Autodesk Inventor part; units mm, degrees
(part 2 of 2)
sketch "Sketch3" plane through (0, 2, 0) normal (0, 1, 0) x (1, 0, 0)
  arc A0 (-46.6476, -62.1619) -> (-47.7526, -62.2283) centre (-47.0018, -65.4919) ccw
  line L0 (-47.7526, -62.2283) -> (-47.7526, -54.9637)
  arc A1 (-46.6476, -56.7523) -> (-47.7526, -54.9637) centre (-48.6476, -56.7523) ccw
  line L1 (-46.1538, -36) -> (-46.1538, -63.7839)
  line L2 (-57.0002, -27.1688) -> (-56.9998, -63.0741)
  line L3 (-56.9998, -63.0741) -> (-59.9998, -63.0742)
  line L4 (-59.9998, -63.0742) -> (-59.9995, -79.762)
  line L5 (-59.9995, -79.762) -> (-57.0005, -79.762)
  line L6 (-57.0005, -79.762) -> (-57.0005, -94.8331)
  line L7 (-57.0005, -94.8331) -> (-41.6794, -94.8331)
  line L8 (-41.6794, -94.8331) -> (-41.6794, -97.8331)
  line L9 (-41.6794, -97.8331) -> (-24.9903, -97.8331)
  line L10 (-24.9903, -97.8331) -> (-24.9903, -94.8331)
  line L11 (-24.9903, -94.8331) -> (24.9903, -94.8331)
  line L12 (24.9903, -94.8331) -> (24.9903, -97.8331)
  line L13 (24.9903, -97.8331) -> (41.6794, -97.8331)
  line L14 (41.6794, -97.8331) -> (41.6794, -94.8331)
  line L15 (41.6794, -94.8331) -> (57.0005, -94.8331)
  line L16 (57.0005, -94.8331) -> (57.0005, -79.762)
  line L17 (57.0005, -79.762) -> (60.0005, -79.762)
  line L18 (60.0005, -79.762) -> (60.0005, -63.0729)
  line L19 (60.0005, -63.0729) -> (57.0005, -63.0729)
  line L20 (57.0005, -63.0729) -> (57.0002, -27.1688)
  line L21 (57.0002, -27.1688) -> (-57.0002, -27.1688)
  circle A2 centre (-10.4999, -30.1712) radius 1
  circle A3 centre (10.5001, -30.1708) radius 1
  circle A4 centre (23.9057, -30.1706) radius 1
  circle A5 centre (44.9057, -30.1702) radius 1
  circle A6 centre (-23.9063, -30.1714) radius 1
  circle A7 centre (-44.9063, -30.1718) radius 1
  circle A8 centre (-47.0018, -34.2919) radius 1.75
  circle A9 centre (28.1782, -34.2919) radius 1.75
  circle A10 centre (28.1782, -65.4919) radius 1.75
  circle A11 centre (-47.0018, -65.4919) radius 1.75
  circle A12 centre (-35.535, -80.373) radius 1.75
  circle A13 centre (34.465, -80.373) radius 1.75
  circle A14 centre (-6.604, -75.238) radius 3
  circle A15 centre (6.604, -75.238) radius 3
  circle A16 centre (-21.844, -75.746) radius 6.43
  circle A17 centre (21.844, -75.746) radius 6.43
  arc A18 (-46.6476, -56.7523) -> (-47.7526, -54.9637) centre (-48.6476, -56.7523) ccw
  line L22 (-46.6476, -56.7523) -> (-46.6476, -62.1619)
  arc A19 (-46.6476, -62.1619) -> (-47.7526, -62.2283) centre (-47.0018, -65.4919) ccw
  line L23 (-46.6476, -68.822) -> (-46.6476, -85.7402)
  arc A20 (-48.6476, -87.7402) -> (-46.6476, -85.7402) centre (-48.6476, -85.7402) ccw
  line L24 (-48.6476, -87.7402) -> (-50.6476, -87.7402)
  arc A21 (-52.6476, -85.7402) -> (-50.6476, -87.7402) centre (-50.6476, -85.7402) ccw
  arc A22 (50.6476, -87.7402) -> (52.6476, -85.7402) centre (50.6476, -85.7402) ccw
  line L25 (50.6476, -87.7402) -> (48.6476, -87.7402)
  arc A23 (46.6476, -85.7402) -> (48.6476, -87.7402) centre (48.6476, -85.7402) ccw
  line L26 (46.6476, -85.7402) -> (46.6476, -56.7523)
  arc A24 (48.6476, -54.7523) -> (46.6476, -56.7523) centre (48.6476, -56.7523) ccw
  line L27 (48.6476, -54.7523) -> (50.6476, -54.7523)
  arc A25 (52.6476, -56.7523) -> (50.6476, -54.7523) centre (50.6476, -56.7523) ccw
  line L28 (52.6476, -56.7523) -> (52.6476, -85.7402)
  line L29 (27.3301, -36) -> (27.3301, -63.7839)
  line L30 (27.3301, -63.7839) -> (-46.1538, -63.7839)
  line L31 (-46.1538, -63.7839) -> (-46.1538, -36)
  line L32 (-46.1538, -36) -> (27.3301, -36)
  line L33 (38.2149, -69.0614) -> (37.21, -69.0614)
  line L34 (37.21, -69.0614) -> (37.21, -65.8232)
  line L35 (37.21, -65.8232) -> (36.0269, -65.8232)
  line L36 (36.0269, -65.8232) -> (36.0269, -65.0614)
  line L37 (36.0269, -65.0614) -> (39.398, -65.0614)
  line L38 (39.398, -65.0614) -> (39.398, -65.8232)
  line L39 (39.398, -65.8232) -> (38.2149, -65.8232)
  line L40 (38.2149, -65.8232) -> (38.2149, -69.0614)
  spline S0 degree 2 poles (39.3883, -54.4407) (39.3883, -55.1798) (38.5423, -55.9739) (37.7124, -55.9739) knots 0 0 0 1 2 2 2
  spline S1 degree 2 poles (37.7124, -55.9739) (36.9053, -55.9739) (36.0366, -55.196) (36.0366, -54.4439) knots 0 0 0 1 2 2 2
  line L41 (36.0366, -54.4439) -> (36.0366, -51.8896)
  line L42 (36.0366, -51.8896) -> (37.0415, -51.8896)
  line L43 (37.0415, -51.8896) -> (37.0415, -54.3856)
  spline S2 degree 2 poles (37.0415, -54.3856) (37.0415, -54.8037) (37.3559, -55.2122) (37.7124, -55.2122) knots 0 0 0 1 2 2 2
  spline S3 degree 2 poles (37.7124, -55.2122) (38.0593, -55.2122) (38.3834, -54.8199) (38.3834, -54.3856) knots 0 0 0 1 2 2 2
  line L44 (38.3834, -54.3856) -> (38.3834, -51.8896)
  line L45 (38.3834, -51.8896) -> (39.3883, -51.8896)
  line L46 (39.3883, -51.8896) -> (39.3883, -54.4407)
  line L47 (32.7825, -86.0448) -> (32.7825, -86.9605)
  line L48 (32.7825, -86.9605) -> (31.5385, -86.9605)
  line L49 (31.5385, -86.9605) -> (31.5385, -86.0448)
  line L50 (31.5385, -86.0448) -> (32.7825, -86.0448)
  spline S4 degree 2 poles (30.5337, -91.0002) (30.2946, -91.1785) (29.6382, -91.373) (29.1803, -91.373) knots 0 0 0 1 2 2 2
  spline S5 degree 2 poles (29.1803, -91.373) (28.7671, -91.373) (28.0256, -91.1906) (27.7825, -91.0691) knots 0 0 0 1 2 2 2
  line L51 (27.7825, -91.0691) -> (27.7825, -90.0764)
  line L52 (27.7825, -90.0764) -> (27.8797, -90.0764)
  spline S6 degree 2 poles (27.8797, -90.0764) (27.9648, -90.1412) (28.1795, -90.2952) (28.37, -90.3803) knots 0 0 0 1 2 2 2
  spline S7 degree 2 poles (28.37, -90.3803) (28.5361, -90.4573) (28.9453, -90.5667) (29.1885, -90.5667) knots 0 0 0 1 2 2 2
  spline S8 degree 2 poles (29.1885, -90.5667) (29.4356, -90.5667) (29.8165, -90.4127) (29.8165, -90.2466) knots 0 0 0 1 2 2 2
  spline S9 degree 2 poles (29.8165, -90.2466) (29.8165, -90.1169) (29.6423, -89.9791) (29.391, -89.9224) knots 0 0 0 1 2 2 2
  spline S10 degree 2 poles (29.391, -89.9224) (29.2573, -89.8859) (28.8481, -89.809) (28.6901, -89.7603) knots 0 0 0 1 2 2 2
  spline S11 degree 2 poles (28.6901, -89.7603) (28.2444, -89.6226) (27.7987, -89.0837) (27.7987, -88.642) knots 0 0 0 1 2 2 2
  spline S12 degree 2 poles (27.7987, -88.642) (27.7987, -88.3908) (28.0296, -87.9451) (28.2565, -87.7709) knots 0 0 0 1 2 2 2
  spline S13 degree 2 poles (28.2565, -87.7709) (28.4794, -87.6007) (29.1398, -87.3981) (29.5572, -87.3981) knots 0 0 0 1 2 2 2
  spline S14 degree 2 poles (29.5572, -87.3981) (29.9543, -87.3981) (30.6188, -87.5561) (30.8457, -87.6655) knots 0 0 0 1 2 2 2
  line L53 (30.8457, -87.6655) -> (30.8457, -88.6218)
  line L54 (30.8457, -88.6218) -> (30.7525, -88.6218)
  spline S15 degree 2 poles (30.7525, -88.6218) (30.6917, -88.5731) (30.4283, -88.4151) (30.3068, -88.3584) knots 0 0 0 1 2 2 2
  spline S16 degree 2 poles (30.3068, -88.3584) (30.1568, -88.2936) (29.7922, -88.2044) (29.6017, -88.2044) knots 0 0 0 1 2 2 2
  spline S17 degree 2 poles (29.6017, -88.2044) (29.3465, -88.2044) (28.994, -88.3786) (28.994, -88.5205) knots 0 0 0 1 2 2 2
  spline S18 degree 2 poles (28.994, -88.5205) (28.994, -88.6501) (29.1682, -88.796) (29.4599, -88.8689) knots 0 0 0 1 2 2 2
  spline S19 degree 2 poles (29.4599, -88.8689) (29.6098, -88.9054) (30.0029, -88.9743) (30.1852, -89.035) knots 0 0 0 1 2 2 2
  spline S20 degree 2 poles (30.1852, -89.035) (30.5904, -89.1647) (31.0118, -89.6712) (31.0118, -90.0926) knots 0 0 0 1 2 2 2
  spline S21 degree 2 poles (31.0118, -90.0926) (31.0118, -90.356) (30.7646, -90.8381) (30.5337, -91.0002) knots 0 0 0 1 2 2 2
  spline S22 degree 2 poles (26.7695, -91.2636) (26.5791, -91.3162) (26.1739, -91.373) (25.8821, -91.373) knots 0 0 0 1 2 2 2
  spline S23 degree 2 poles (25.8821, -91.373) (24.8124, -91.373) (23.6739, -90.3519) (23.6739, -89.4078) knots 0 0 0 1 2 2 2
  spline S24 degree 2 poles (23.6739, -89.4078) (23.6739, -88.484) (24.7355, -87.3819) (25.6917, -87.3819) knots 0 0 0 1 2 2 2
  spline S25 degree 2 poles (25.6917, -87.3819) (26.5547, -87.3819) (27.4299, -88.3179) (27.4299, -89.185) knots 0 0 0 1 2 2 2
  line L55 (27.4299, -89.185) -> (27.4299, -89.6104)
  line L56 (27.4299, -89.6104) -> (24.8489, -89.6104)
  spline S26 degree 2 poles (24.8489, -89.6104) (24.8651, -89.8738) (25.0555, -90.2222) (25.2095, -90.3276) knots 0 0 0 1 2 2 2
  spline S27 degree 2 poles (25.2095, -90.3276) (25.3594, -90.4329) (25.7646, -90.5221) (26.0037, -90.5221) knots 0 0 0 1 2 2 2
  spline S28 degree 2 poles (26.0037, -90.5221) (26.2063, -90.5221) (26.6034, -90.4329) (26.7695, -90.356) knots 0 0 0 1 2 2 2
  spline S29 degree 2 poles (26.7695, -90.356) (26.9154, -90.2952) (27.1585, -90.1453) (27.2355, -90.0885) knots 0 0 0 1 2 2 2
  line L57 (27.2355, -90.0885) -> (27.3611, -90.0885)
  line L58 (27.3611, -90.0885) -> (27.3611, -91.061)
  spline S30 degree 2 poles (27.3611, -91.061) (27.2152, -91.1177) (26.9802, -91.215) (26.7695, -91.2636) knots 0 0 0 1 2 2 2
  line L59 (10.1082, -88.8162) -> (10.1082, -91.2717)
  line L60 (10.1082, -91.2717) -> (8.9251, -91.2717)
  line L61 (8.9251, -91.2717) -> (8.9251, -89.4038)
  spline S31 degree 2 poles (8.9251, -89.4038) (8.9251, -89.1728) (8.8886, -88.719) (8.84, -88.6137) knots 0 0 0 1 2 2 2
  spline S32 degree 2 poles (8.84, -88.6137) (8.7792, -88.484) (8.5523, -88.3746) (8.3578, -88.3746) knots 0 0 0 1 2 2 2
  spline S33 degree 2 poles (8.3578, -88.3746) (8.216, -88.3746) (7.9202, -88.484) (7.7541, -88.6015) knots 0 0 0 1 2 2 2
  line L62 (7.7541, -88.6015) -> (7.7541, -91.2717)
  line L63 (7.7541, -91.2717) -> (6.5791, -91.2717)
  line L64 (6.5791, -91.2717) -> (6.5791, -87.4994)
  line L65 (6.5791, -87.4994) -> (7.7541, -87.4994)
  line L66 (7.7541, -87.4994) -> (7.7541, -87.9167)
  spline S34 degree 2 poles (7.7541, -87.9167) (8.0418, -87.6736) (8.5888, -87.3981) (8.921, -87.3981) knots 0 0 0 1 2 2 2
  spline S35 degree 2 poles (8.921, -87.3981) (9.4964, -87.3981) (10.1082, -88.1274) (10.1082, -88.8162) knots 0 0 0 1 2 2 2
  spline S36 degree 2 poles (0.2055, -91.0002) (-0.0336, -91.1785) (-0.69, -91.373) (-1.1479, -91.373) knots 0 0 0 1 2 2 2
  spline S37 degree 2 poles (-1.1479, -91.373) (-1.5611, -91.373) (-2.3026, -91.1906) (-2.5457, -91.0691) knots 0 0 0 1 2 2 2
  line L67 (-2.5457, -91.0691) -> (-2.5457, -90.0764)
  line L68 (-2.5457, -90.0764) -> (-2.4485, -90.0764)
  spline S38 degree 2 poles (-2.4485, -90.0764) (-2.3634, -90.1412) (-2.1487, -90.2952) (-1.9582, -90.3803) knots 0 0 0 1 2 2 2
  spline S39 degree 2 poles (-1.9582, -90.3803) (-1.7921, -90.4573) (-1.3829, -90.5667) (-1.1398, -90.5667) knots 0 0 0 1 2 2 2
  spline S40 degree 2 poles (-1.1398, -90.5667) (-0.8926, -90.5667) (-0.5117, -90.4127) (-0.5117, -90.2466) knots 0 0 0 1 2 2 2
  spline S41 degree 2 poles (-0.5117, -90.2466) (-0.5117, -90.1169) (-0.6859, -89.9791) (-0.9372, -89.9224) knots 0 0 0 1 2 2 2
  spline S42 degree 2 poles (-0.9372, -89.9224) (-1.0709, -89.8859) (-1.4801, -89.809) (-1.6381, -89.7603) knots 0 0 0 1 2 2 2
  spline S43 degree 2 poles (-1.6381, -89.7603) (-2.0838, -89.6226) (-2.5295, -89.0837) (-2.5295, -88.642) knots 0 0 0 1 2 2 2
  spline S44 degree 2 poles (-2.5295, -88.642) (-2.5295, -88.3908) (-2.2986, -87.9451) (-2.0717, -87.7709) knots 0 0 0 1 2 2 2
  spline S45 degree 2 poles (-2.0717, -87.7709) (-1.8488, -87.6007) (-1.1884, -87.3981) (-0.771, -87.3981) knots 0 0 0 1 2 2 2
  spline S46 degree 2 poles (-0.771, -87.3981) (-0.3739, -87.3981) (0.2906, -87.5561) (0.5175, -87.6655) knots 0 0 0 1 2 2 2
  line L69 (0.5175, -87.6655) -> (0.5175, -88.6218)
  line L70 (0.5175, -88.6218) -> (0.4243, -88.6218)
  spline S47 degree 2 poles (0.4243, -88.6218) (0.3635, -88.5731) (0.1001, -88.4151) (-0.0214, -88.3584) knots 0 0 0 1 2 2 2
  spline S48 degree 2 poles (-0.0214, -88.3584) (-0.1714, -88.2936) (-0.536, -88.2044) (-0.7265, -88.2044) knots 0 0 0 1 2 2 2
  spline S49 degree 2 poles (-0.7265, -88.2044) (-0.9817, -88.2044) (-1.3342, -88.3786) (-1.3342, -88.5205) knots 0 0 0 1 2 2 2
  spline S50 degree 2 poles (-1.3342, -88.5205) (-1.3342, -88.6501) (-1.16, -88.796) (-0.8683, -88.8689) knots 0 0 0 1 2 2 2
  spline S51 degree 2 poles (-0.8683, -88.8689) (-0.7184, -88.9054) (-0.3253, -88.9743) (-0.143, -89.035) knots 0 0 0 1 2 2 2
  spline S52 degree 2 poles (-0.143, -89.035) (0.2622, -89.1647) (0.6836, -89.6712) (0.6836, -90.0926) knots 0 0 0 1 2 2 2
  spline S53 degree 2 poles (0.6836, -90.0926) (0.6836, -90.356) (0.4364, -90.8381) (0.2055, -91.0002) knots 0 0 0 1 2 2 2
  line L71 (-4.3326, -91.2717) -> (-4.3326, -90.8705)
  spline S54 degree 2 poles (-4.3326, -90.8705) (-4.4542, -90.9718) (-4.6446, -91.1339) (-4.8067, -91.215) knots 0 0 0 1 2 2 2
  spline S55 degree 2 poles (-4.8067, -91.215) (-4.9647, -91.2919) (-5.2645, -91.373) (-5.532, -91.373) knots 0 0 0 1 2 2 2
  spline S56 degree 2 poles (-5.532, -91.373) (-6.0344, -91.373) (-6.6949, -90.7004) (-6.6949, -90.1898) knots 0 0 0 1 2 2 2
  spline S57 degree 2 poles (-6.6949, -90.1898) (-6.6949, -89.7725) (-6.3586, -89.2538) (-6.0425, -89.1039) knots 0 0 0 1 2 2 2
  spline S58 degree 2 poles (-6.0425, -89.1039) (-5.7224, -88.95) (-4.8351, -88.8284) (-4.3245, -88.796) knots 0 0 0 1 2 2 2
  line L72 (-4.3245, -88.796) -> (-4.3245, -88.7757)
  spline S59 degree 2 poles (-4.3245, -88.7757) (-4.3245, -88.4637) (-4.7864, -88.2247) (-5.2483, -88.2247) knots 0 0 0 1 2 2 2
  spline S60 degree 2 poles (-5.2483, -88.2247) (-5.455, -88.2247) (-6.0141, -88.3746) (-6.2775, -88.4921) knots 0 0 0 1 2 2 2
  line L73 (-6.2775, -88.4921) -> (-6.3788, -88.4921)
  line L74 (-6.3788, -88.4921) -> (-6.3788, -87.5804)
  spline S61 degree 2 poles (-6.3788, -87.5804) (-6.2046, -87.5318) (-5.4266, -87.394) (-5.0295, -87.394) knots 0 0 0 1 2 2 2
  spline S62 degree 2 poles (-5.0295, -87.394) (-4.0571, -87.394) (-3.1657, -88.0423) (-3.1657, -88.7068) knots 0 0 0 1 2 2 2
  line L75 (-3.1657, -88.7068) -> (-3.1657, -91.2717)
  line L76 (-3.1657, -91.2717) -> (-4.3326, -91.2717)
  line L77 (-10.1308, -86.0448) -> (-10.1308, -86.9605)
  line L78 (-10.1308, -86.9605) -> (-11.3748, -86.9605)
  line L79 (-11.3748, -86.9605) -> (-11.3748, -86.0448)
  line L80 (-11.3748, -86.0448) -> (-10.1308, -86.0448)
  spline S63 degree 2 poles (-12.3796, -91.0002) (-12.6187, -91.1785) (-13.2751, -91.373) (-13.7329, -91.373) knots 0 0 0 1 2 2 2
  spline S64 degree 2 poles (-13.7329, -91.373) (-14.1462, -91.373) (-14.8877, -91.1906) (-15.1308, -91.0691) knots 0 0 0 1 2 2 2
  line L81 (-15.1308, -91.0691) -> (-15.1308, -90.0764)
  line L82 (-15.1308, -90.0764) -> (-15.0336, -90.0764)
  spline S65 degree 2 poles (-15.0336, -90.0764) (-14.9485, -90.1412) (-14.7338, -90.2952) (-14.5433, -90.3803) knots 0 0 0 1 2 2 2
  spline S66 degree 2 poles (-14.5433, -90.3803) (-14.3772, -90.4573) (-13.968, -90.5667) (-13.7248, -90.5667) knots 0 0 0 1 2 2 2
  spline S67 degree 2 poles (-13.7248, -90.5667) (-13.4777, -90.5667) (-13.0968, -90.4127) (-13.0968, -90.2466) knots 0 0 0 1 2 2 2
  spline S68 degree 2 poles (-13.0968, -90.2466) (-13.0968, -90.1169) (-13.271, -89.9791) (-13.5222, -89.9224) knots 0 0 0 1 2 2 2
  spline S69 degree 2 poles (-13.5222, -89.9224) (-13.656, -89.8859) (-14.0652, -89.809) (-14.2232, -89.7603) knots 0 0 0 1 2 2 2
  spline S70 degree 2 poles (-14.2232, -89.7603) (-14.6689, -89.6226) (-15.1146, -89.0837) (-15.1146, -88.642) knots 0 0 0 1 2 2 2
  spline S71 degree 2 poles (-15.1146, -88.642) (-15.1146, -88.3908) (-14.8837, -87.9451) (-14.6568, -87.7709) knots 0 0 0 1 2 2 2
  spline S72 degree 2 poles (-14.6568, -87.7709) (-14.4339, -87.6007) (-13.7735, -87.3981) (-13.3561, -87.3981) knots 0 0 0 1 2 2 2
  spline S73 degree 2 poles (-13.3561, -87.3981) (-12.959, -87.3981) (-12.2945, -87.5561) (-12.0676, -87.6655) knots 0 0 0 1 2 2 2
  line L83 (-12.0676, -87.6655) -> (-12.0676, -88.6218)
  line L84 (-12.0676, -88.6218) -> (-12.1608, -88.6218)
  spline S74 degree 2 poles (-12.1608, -88.6218) (-12.2216, -88.5731) (-12.485, -88.4151) (-12.6065, -88.3584) knots 0 0 0 1 2 2 2
  spline S75 degree 2 poles (-12.6065, -88.3584) (-12.7564, -88.2936) (-13.1211, -88.2044) (-13.3115, -88.2044) knots 0 0 0 1 2 2 2
  spline S76 degree 2 poles (-13.3115, -88.2044) (-13.5668, -88.2044) (-13.9193, -88.3786) (-13.9193, -88.5205) knots 0 0 0 1 2 2 2
  spline S77 degree 2 poles (-13.9193, -88.5205) (-13.9193, -88.6501) (-13.7451, -88.796) (-13.4534, -88.8689) knots 0 0 0 1 2 2 2
  spline S78 degree 2 poles (-13.4534, -88.8689) (-13.3034, -88.9054) (-12.9104, -88.9743) (-12.7281, -89.035) knots 0 0 0 1 2 2 2
  spline S79 degree 2 poles (-12.7281, -89.035) (-12.3229, -89.1647) (-11.9015, -89.6712) (-11.9015, -90.0926) knots 0 0 0 1 2 2 2
  spline S80 degree 2 poles (-11.9015, -90.0926) (-11.9015, -90.356) (-12.1487, -90.8381) (-12.3796, -91.0002) knots 0 0 0 1 2 2 2
  line L85 (-23.6073, -87.4994) -> (-22.3958, -87.4994)
  line L86 (-22.3958, -87.4994) -> (-23.7492, -91.2717)
  line L87 (-23.7492, -91.2717) -> (-25.0336, -91.2717)
  line L88 (-25.0336, -91.2717) -> (-26.3748, -87.4994)
  line L89 (-26.3748, -87.4994) -> (-25.1389, -87.4994)
  line L90 (-25.1389, -87.4994) -> (-24.3691, -89.9913)
  line L91 (-24.3691, -89.9913) -> (-23.6073, -87.4994)
  line L92 (-26.8245, -87.4994) -> (-26.8245, -91.2717)
  line L93 (-26.8245, -91.2717) -> (-27.9996, -91.2717)
  line L94 (-27.9996, -91.2717) -> (-27.9996, -87.4994)
  line L95 (-27.9996, -87.4994) -> (-26.8245, -87.4994)
  spline S81 degree 2 poles (-33.2953, -89.4605) (-33.2953, -90.3843) (-34.3529, -91.377) (-35.3902, -91.377) knots 0 0 0 1 2 2 2
  spline S82 degree 2 poles (-35.3902, -91.377) (-36.3991, -91.377) (-37.485, -90.4046) (-37.485, -89.4645) knots 0 0 0 1 2 2 2
  line L96 (-37.485, -89.4645) -> (-37.485, -86.2717)
  line L97 (-37.485, -86.2717) -> (-36.2289, -86.2717)
  line L98 (-36.2289, -86.2717) -> (-36.2289, -89.3916)
  spline S83 degree 2 poles (-36.2289, -89.3916) (-36.2289, -89.9143) (-35.8359, -90.4248) (-35.3902, -90.4248) knots 0 0 0 1 2 2 2
  spline S84 degree 2 poles (-35.3902, -90.4248) (-34.9566, -90.4248) (-34.5514, -89.9346) (-34.5514, -89.3916) knots 0 0 0 1 2 2 2
  line L99 (-34.5514, -89.3916) -> (-34.5514, -86.2717)
  line L100 (-34.5514, -86.2717) -> (-33.2953, -86.2717)
  line L101 (-33.2953, -86.2717) -> (-33.2953, -89.4605)
  line L102 (-28.8707, -88.8162) -> (-28.8707, -91.2717)
  line L103 (-28.8707, -91.2717) -> (-30.0539, -91.2717)
  line L104 (-30.0539, -91.2717) -> (-30.0539, -89.4038)
  spline S85 degree 2 poles (-30.0539, -89.4038) (-30.0539, -89.1728) (-30.0903, -88.719) (-30.1389, -88.6137) knots 0 0 0 1 2 2 2
  spline S86 degree 2 poles (-30.1389, -88.6137) (-30.1997, -88.484) (-30.4266, -88.3746) (-30.6211, -88.3746) knots 0 0 0 1 2 2 2
  spline S87 degree 2 poles (-30.6211, -88.3746) (-30.7629, -88.3746) (-31.0587, -88.484) (-31.2248, -88.6015) knots 0 0 0 1 2 2 2
  line L105 (-31.2248, -88.6015) -> (-31.2248, -91.2717)
  line L106 (-31.2248, -91.2717) -> (-32.3999, -91.2717)
  line L107 (-32.3999, -91.2717) -> (-32.3999, -87.4994)
  line L108 (-32.3999, -87.4994) -> (-31.2248, -87.4994)
  line L109 (-31.2248, -87.4994) -> (-31.2248, -87.9167)
  spline S88 degree 2 poles (-31.2248, -87.9167) (-30.9372, -87.6736) (-30.3902, -87.3981) (-30.0579, -87.3981) knots 0 0 0 1 2 2 2
  spline S89 degree 2 poles (-30.0579, -87.3981) (-29.4825, -87.3981) (-28.8707, -88.1274) (-28.8707, -88.8162) knots 0 0 0 1 2 2 2
  line L110 (-26.788, -86.0448) -> (-26.788, -86.9605)
  line L111 (-26.788, -86.9605) -> (-28.032, -86.9605)
  line L112 (-28.032, -86.9605) -> (-28.032, -86.0448)
  line L113 (-28.032, -86.0448) -> (-26.788, -86.0448)
  spline S90 degree 2 poles (-19.126, -91.2636) (-19.3164, -91.3162) (-19.7216, -91.373) (-20.0133, -91.373) knots 0 0 0 1 2 2 2
  spline S91 degree 2 poles (-20.0133, -91.373) (-21.083, -91.373) (-22.2216, -90.3519) (-22.2216, -89.4078) knots 0 0 0 1 2 2 2
  spline S92 degree 2 poles (-22.2216, -89.4078) (-22.2216, -88.484) (-21.16, -87.3819) (-20.2038, -87.3819) knots 0 0 0 1 2 2 2
  spline S93 degree 2 poles (-20.2038, -87.3819) (-19.3407, -87.3819) (-18.4655, -88.3179) (-18.4655, -89.185) knots 0 0 0 1 2 2 2
  line L114 (-18.4655, -89.185) -> (-18.4655, -89.6104)
  line L115 (-18.4655, -89.6104) -> (-21.0466, -89.6104)
  spline S94 degree 2 poles (-21.0466, -89.6104) (-21.0303, -89.8738) (-20.8399, -90.2222) (-20.6859, -90.3276) knots 0 0 0 1 2 2 2
  spline S95 degree 2 poles (-20.6859, -90.3276) (-20.536, -90.4329) (-20.1308, -90.5221) (-19.8918, -90.5221) knots 0 0 0 1 2 2 2
  spline S96 degree 2 poles (-19.8918, -90.5221) (-19.6892, -90.5221) (-19.2921, -90.4329) (-19.126, -90.356) knots 0 0 0 1 2 2 2
  spline S97 degree 2 poles (-19.126, -90.356) (-18.9801, -90.2952) (-18.737, -90.1453) (-18.66, -90.0885) knots 0 0 0 1 2 2 2
  line L116 (-18.66, -90.0885) -> (-18.5344, -90.0885)
  line L117 (-18.5344, -90.0885) -> (-18.5344, -91.061)
  spline S98 degree 2 poles (-18.5344, -91.061) (-18.6803, -91.1177) (-18.9153, -91.215) (-19.126, -91.2636) knots 0 0 0 1 2 2 2
  line L118 (-15.3294, -87.4994) -> (-15.3294, -88.6137)
  line L119 (-15.3294, -88.6137) -> (-15.4266, -88.6137)
  spline S99 degree 2 poles (-15.4266, -88.6137) (-15.4955, -88.5893) (-15.7508, -88.565) (-15.9047, -88.565) knots 0 0 0 1 2 2 2
  spline S100 degree 2 poles (-15.9047, -88.565) (-16.0871, -88.565) (-16.4963, -88.6744) (-16.6868, -88.7474) knots 0 0 0 1 2 2 2
  line L120 (-16.6868, -88.7474) -> (-16.6868, -91.2717)
  line L121 (-16.6868, -91.2717) -> (-17.8618, -91.2717)
  line L122 (-17.8618, -91.2717) -> (-17.8618, -87.4994)
  line L123 (-17.8618, -87.4994) -> (-16.6868, -87.4994)
  line L124 (-16.6868, -87.4994) -> (-16.6868, -88.0423)
  spline S101 degree 2 poles (-16.6868, -88.0423) (-16.6057, -87.9694) (-16.3221, -87.7425) (-16.2046, -87.6736) knots 0 0 0 1 2 2 2
  spline S102 degree 2 poles (-16.2046, -87.6736) (-16.0749, -87.5966) (-15.7346, -87.4872) (-15.5846, -87.4872) knots 0 0 0 1 2 2 2
  spline S103 degree 2 poles (-15.5846, -87.4872) (-15.5279, -87.4872) (-15.3861, -87.4953) (-15.3294, -87.4994) knots 0 0 0 1 2 2 2
  line L125 (-10.1673, -87.4994) -> (-10.1673, -91.2717)
  line L126 (-10.1673, -91.2717) -> (-11.3423, -91.2717)
  line L127 (-11.3423, -91.2717) -> (-11.3423, -87.4994)
  line L128 (-11.3423, -87.4994) -> (-10.1673, -87.4994)
  spline S104 degree 2 poles (-6.8893, -91.2393) (-7.0798, -91.2879) (-7.5093, -91.3446) (-7.8253, -91.3446) knots 0 0 0 1 2 2 2
  spline S105 degree 2 poles (-7.8253, -91.3446) (-8.5425, -91.3446) (-9.1989, -90.753) (-9.1989, -90.0804) knots 0 0 0 1 2 2 2
  line L129 (-9.1989, -90.0804) -> (-9.1989, -88.3179)
  line L130 (-9.1989, -88.3179) -> (-9.6487, -88.3179)
  line L131 (-9.6487, -88.3179) -> (-9.6487, -87.4994)
  line L132 (-9.6487, -87.4994) -> (-9.1989, -87.4994)
  line L133 (-9.1989, -87.4994) -> (-9.1989, -86.4216)
  line L134 (-9.1989, -86.4216) -> (-8.0239, -86.4216)
  line L135 (-8.0239, -86.4216) -> (-8.0239, -87.4994)
  line L136 (-8.0239, -87.4994) -> (-6.8893, -87.4994)
  line L137 (-6.8893, -87.4994) -> (-6.8893, -88.3179)
  line L138 (-6.8893, -88.3179) -> (-8.0239, -88.3179)
  line L139 (-8.0239, -88.3179) -> (-8.0239, -89.659)
  spline S106 degree 2 poles (-8.0239, -89.659) (-8.0239, -89.8576) (-8.0158, -90.1534) (-7.9671, -90.2709) knots 0 0 0 1 2 2 2
  spline S107 degree 2 poles (-7.9671, -90.2709) (-7.9185, -90.3884) (-7.6795, -90.5261) (-7.4526, -90.5261) knots 0 0 0 1 2 2 2
  spline S108 degree 2 poles (-7.4526, -90.5261) (-7.3553, -90.5261) (-7.0514, -90.4451) (-6.9906, -90.4127) knots 0 0 0 1 2 2 2
  line L140 (-6.9906, -90.4127) -> (-6.8893, -90.4127)
  line L141 (-6.8893, -90.4127) -> (-6.8893, -91.2393)
  line L142 (5.8132, -90.4005) -> (5.8132, -91.2717)
  line L143 (5.8132, -91.2717) -> (3.1228, -91.2717)
  line L144 (3.1228, -91.2717) -> (3.1228, -90.4005)
  line L145 (3.1228, -90.4005) -> (3.84, -90.4005)
  line L146 (3.84, -90.4005) -> (3.84, -87.1428)
  line L147 (3.84, -87.1428) -> (3.1228, -87.1428)
  line L148 (3.1228, -87.1428) -> (3.1228, -86.2717)
  line L149 (3.1228, -86.2717) -> (5.8132, -86.2717)
  line L150 (5.8132, -86.2717) -> (5.8132, -87.1428)
  line L151 (5.8132, -87.1428) -> (5.0961, -87.1428)
  line L152 (5.0961, -87.1428) -> (5.0961, -90.4005)
  line L153 (5.0961, -90.4005) -> (5.8132, -90.4005)
  line L154 (14.4073, -86.0488) -> (14.4073, -91.2717)
  line L155 (14.4073, -91.2717) -> (13.2322, -91.2717)
  line L156 (13.2322, -91.2717) -> (13.2322, -90.8786)
  spline S109 degree 2 poles (13.2322, -90.8786) (13.1188, -90.9718) (12.827, -91.1866) (12.7136, -91.2433) knots 0 0 0 1 2 2 2
  spline S110 degree 2 poles (12.7136, -91.2433) (12.5758, -91.3081) (12.3003, -91.377) (12.1098, -91.377) knots 0 0 0 1 2 2 2
  spline S111 degree 2 poles (12.1098, -91.377) (11.4656, -91.377) (10.712, -90.3073) (10.712, -89.4159) knots 0 0 0 1 2 2 2
  spline S112 degree 2 poles (10.712, -89.4159) (10.712, -88.9216) (10.9672, -88.1963) (11.1901, -87.9289) knots 0 0 0 1 2 2 2
  spline S113 degree 2 poles (11.1901, -87.9289) (11.3967, -87.6817) (11.9802, -87.3981) (12.3043, -87.3981) knots 0 0 0 1 2 2 2
  spline S114 degree 2 poles (12.3043, -87.3981) (12.6001, -87.3981) (12.981, -87.5237) (13.2322, -87.6534) knots 0 0 0 1 2 2 2
  line L157 (13.2322, -87.6534) -> (13.2322, -86.0488)
  line L158 (13.2322, -86.0488) -> (14.4073, -86.0488)
  spline S115 degree 2 poles (16.9802, -87.3819) (17.904, -87.3819) (18.9251, -88.4516) (18.9251, -89.3876) knots 0 0 0 1 2 2 2
  spline S116 degree 2 poles (18.9251, -89.3876) (18.9251, -90.3195) (17.9081, -91.3892) (16.9802, -91.3892) knots 0 0 0 1 2 2 2
  spline S117 degree 2 poles (16.9802, -91.3892) (16.0564, -91.3892) (15.0312, -90.3195) (15.0312, -89.3876) knots 0 0 0 1 2 2 2
  spline S118 degree 2 poles (15.0312, -89.3876) (15.0312, -88.4475) (16.0564, -87.3819) (16.9802, -87.3819) knots 0 0 0 1 2 2 2
  line L159 (23.0782, -88.8162) -> (23.0782, -91.2717)
  line L160 (23.0782, -91.2717) -> (21.8951, -91.2717)
  line L161 (21.8951, -91.2717) -> (21.8951, -89.4038)
  spline S119 degree 2 poles (21.8951, -89.4038) (21.8951, -89.1728) (21.8586, -88.719) (21.81, -88.6137) knots 0 0 0 1 2 2 2
  spline S120 degree 2 poles (21.81, -88.6137) (21.7492, -88.484) (21.5223, -88.3746) (21.3278, -88.3746) knots 0 0 0 1 2 2 2
  spline S121 degree 2 poles (21.3278, -88.3746) (21.186, -88.3746) (20.8902, -88.484) (20.7241, -88.6015) knots 0 0 0 1 2 2 2
  line L162 (20.7241, -88.6015) -> (20.7241, -91.2717)
  line L163 (20.7241, -91.2717) -> (19.5491, -91.2717)
  line L164 (19.5491, -91.2717) -> (19.5491, -87.4994)
  line L165 (19.5491, -87.4994) -> (20.7241, -87.4994)
  line L166 (20.7241, -87.4994) -> (20.7241, -87.9167)
  spline S122 degree 2 poles (20.7241, -87.9167) (21.0118, -87.6736) (21.5588, -87.3981) (21.891, -87.3981) knots 0 0 0 1 2 2 2
  spline S123 degree 2 poles (21.891, -87.3981) (22.4664, -87.3981) (23.0782, -88.1274) (23.0782, -88.8162) knots 0 0 0 1 2 2 2
  line L167 (32.746, -87.4994) -> (32.746, -91.2717)
  line L168 (32.746, -91.2717) -> (31.5709, -91.2717)
  line L169 (31.5709, -91.2717) -> (31.5709, -87.4994)
  line L170 (31.5709, -87.4994) -> (32.746, -87.4994)
  line L171 (35.7241, -91.2717) -> (35.7241, -90.8705)
  spline S124 degree 2 poles (35.7241, -90.8705) (35.6026, -90.9718) (35.4121, -91.1339) (35.25, -91.215) knots 0 0 0 1 2 2 2
  spline S125 degree 2 poles (35.25, -91.215) (35.092, -91.2919) (34.7922, -91.373) (34.5248, -91.373) knots 0 0 0 1 2 2 2
  spline S126 degree 2 poles (34.5248, -91.373) (34.0223, -91.373) (33.3619, -90.7004) (33.3619, -90.1898) knots 0 0 0 1 2 2 2
  spline S127 degree 2 poles (33.3619, -90.1898) (33.3619, -89.7725) (33.6982, -89.2538) (34.0142, -89.1039) knots 0 0 0 1 2 2 2
  spline S128 degree 2 poles (34.0142, -89.1039) (34.3343, -88.95) (35.2217, -88.8284) (35.7322, -88.796) knots 0 0 0 1 2 2 2
  line L172 (35.7322, -88.796) -> (35.7322, -88.7757)
  spline S129 degree 2 poles (35.7322, -88.7757) (35.7322, -88.4637) (35.2703, -88.2247) (34.8084, -88.2247) knots 0 0 0 1 2 2 2
  spline S130 degree 2 poles (34.8084, -88.2247) (34.6017, -88.2247) (34.0426, -88.3746) (33.7792, -88.4921) knots 0 0 0 1 2 2 2
  line L173 (33.7792, -88.4921) -> (33.6779, -88.4921)
  line L174 (33.6779, -88.4921) -> (33.6779, -87.5804)
  spline S131 degree 2 poles (33.6779, -87.5804) (33.8521, -87.5318) (34.6301, -87.394) (35.0272, -87.394) knots 0 0 0 1 2 2 2
  spline S132 degree 2 poles (35.0272, -87.394) (35.9996, -87.394) (36.891, -88.0423) (36.891, -88.7068) knots 0 0 0 1 2 2 2
  line L175 (36.891, -88.7068) -> (36.891, -91.2717)
  line L176 (36.891, -91.2717) -> (35.7241, -91.2717)
  line L177 (38.4807, -34.4302) -> (39.8259, -36.132)
  line L178 (39.8259, -36.132) -> (38.6039, -36.132)
  line L179 (38.6039, -36.132) -> (37.492, -34.6636)
  line L180 (37.492, -34.6636) -> (37.129, -34.6636)
  line L181 (37.129, -34.6636) -> (37.129, -36.132)
  line L182 (37.129, -36.132) -> (36.1306, -36.132)
  line L183 (36.1306, -36.132) -> (36.1306, -32.132)
  line L184 (36.1306, -32.132) -> (37.7384, -32.132)
  spline S133 degree 2 poles (37.7384, -32.132) (38.0722, -32.132) (38.565, -32.2162) (38.7757, -32.3459) knots 0 0 0 1 2 2 2
  spline S134 degree 2 poles (38.7757, -32.3459) (38.9896, -32.482) (39.2424, -32.9067) (39.2424, -33.2308) knots 0 0 0 1 2 2 2
  spline S135 degree 2 poles (39.2424, -33.2308) (39.2424, -33.6879) (38.8275, -34.2616) (38.4807, -34.4302) knots 0 0 0 1 2 2 2
  spline S136 degree 2 poles (37.7108, -38.6336) (38.612, -38.6336) (39.6492, -39.7486) (39.6492, -40.7179) knots 0 0 0 1 2 2 2
  spline S137 degree 2 poles (39.6492, -40.7179) (39.6492, -41.6903) (38.612, -42.8021) (37.7108, -42.8021) knots 0 0 0 1 2 2 2
  spline S138 degree 2 poles (37.7108, -42.8021) (36.8064, -42.8021) (35.7757, -41.6773) (35.7757, -40.7179) knots 0 0 0 1 2 2 2
  spline S139 degree 2 poles (35.7757, -40.7179) (35.7757, -39.7551) (36.8064, -38.6336) (37.7108, -38.6336) knots 0 0 0 1 2 2 2
  spline S140 degree 2 poles (38.6201, -47.1093) (38.9928, -47.1871) (39.4369, -47.67) (39.4369, -48.0785) knots 0 0 0 1 2 2 2
  spline S141 degree 2 poles (39.4369, -48.0785) (39.4369, -48.3767) (39.21, -48.8272) (39.022, -48.9764) knots 0 0 0 1 2 2 2
  spline S142 degree 2 poles (39.022, -48.9764) (38.7951, -49.1546) (38.257, -49.3037) (37.8389, -49.3037) knots 0 0 0 1 2 2 2
  line L185 (37.8389, -49.3037) -> (36.2408, -49.3037)
  line L186 (36.2408, -49.3037) -> (36.2408, -45.3037)
  line L187 (36.2408, -45.3037) -> (37.6509, -45.3037)
  spline S143 degree 2 poles (37.6509, -45.3037) (38.0917, -45.3037) (38.5455, -45.3718) (38.7432, -45.4788) knots 0 0 0 1 2 2 2
  spline S144 degree 2 poles (38.7432, -45.4788) (38.9604, -45.5922) (39.1711, -45.9812) (39.1711, -46.2341) knots 0 0 0 1 2 2 2
  spline S145 degree 2 poles (39.1711, -46.2341) (39.1711, -46.5258) (38.8794, -46.9828) (38.6201, -47.0898) knots 0 0 0 1 2 2 2
  line L188 (38.6201, -47.0898) -> (38.6201, -47.1093)
  spline S146 degree 2 poles (39.3543, -61.2243) (39.3543, -61.8208) (38.4175, -62.5468) (37.6201, -62.5468) knots 0 0 0 1 2 2 2
  spline S147 degree 2 poles (37.6201, -62.5468) (37.1598, -62.5468) (36.4661, -62.3686) (36.1679, -62.2389) knots 0 0 0 1 2 2 2
  line L189 (36.1679, -62.2389) -> (36.1679, -61.2859)
  line L190 (36.1679, -61.2859) -> (36.2586, -61.2859)
  spline S148 degree 2 poles (36.2586, -61.2859) (36.5601, -61.542) (37.2829, -61.8175) (37.6233, -61.8175) knots 0 0 0 1 2 2 2
  spline S149 degree 2 poles (37.6233, -61.8175) (37.7108, -61.8175) (37.9928, -61.7786) (38.0771, -61.7397) knots 0 0 0 1 2 2 2
  spline S150 degree 2 poles (38.0771, -61.7397) (38.1808, -61.6943) (38.3267, -61.529) (38.3267, -61.3961) knots 0 0 0 1 2 2 2
  spline S151 degree 2 poles (38.3267, -61.3961) (38.3267, -61.2438) (38.0901, -61.0558) (37.928, -61.0136) knots 0 0 0 1 2 2 2
  spline S152 degree 2 poles (37.928, -61.0136) (37.7238, -60.9585) (37.2603, -60.8645) (37.056, -60.7932) knots 0 0 0 1 2 2 2
  spline S153 degree 2 poles (37.056, -60.7932) (36.5925, -60.6311) (36.1906, -60.0768) (36.1906, -59.6619) knots 0 0 0 1 2 2 2
  spline S154 degree 2 poles (36.1906, -59.6619) (36.1906, -59.1011) (37.1403, -58.4042) (37.8534, -58.4042) knots 0 0 0 1 2 2 2
  spline S155 degree 2 poles (37.8534, -58.4042) (38.21, -58.4042) (38.9167, -58.5501) (39.1954, -58.6733) knots 0 0 0 1 2 2 2
  line L191 (39.1954, -58.6733) -> (39.1954, -59.5874)
  line L192 (39.1954, -59.5874) -> (39.1079, -59.5874)
  spline S156 degree 2 poles (39.1079, -59.5874) (38.8842, -59.3961) (38.2424, -59.1336) (37.9053, -59.1336) knots 0 0 0 1 2 2 2
  spline S157 degree 2 poles (37.9053, -59.1336) (37.7724, -59.1336) (37.565, -59.1725) (37.4483, -59.2243) knots 0 0 0 1 2 2 2
  spline S158 degree 2 poles (37.4483, -59.2243) (37.3543, -59.2665) (37.2181, -59.435) (37.2181, -59.5387) knots 0 0 0 1 2 2 2
  spline S159 degree 2 poles (37.2181, -59.5387) (37.2181, -59.6943) (37.4353, -59.8726) (37.7465, -59.9439) knots 0 0 0 1 2 2 2
  spline S160 degree 2 poles (37.7465, -59.9439) (37.9475, -59.9893) (38.3202, -60.0768) (38.5342, -60.1514) knots 0 0 0 1 2 2 2
  spline S161 degree 2 poles (38.5342, -60.1514) (38.9491, -60.3037) (39.3543, -60.8094) (39.3543, -61.2243) knots 0 0 0 1 2 2 2
  line L193 (36.8016, -75.6473) -> (35.7967, -75.6473)
  line L194 (35.7967, -75.6473) -> (37.1484, -71.6473)
  line L195 (37.1484, -71.6473) -> (38.244, -71.6473)
  line L196 (38.244, -71.6473) -> (39.5957, -75.6473)
  line L197 (39.5957, -75.6473) -> (38.5617, -75.6473)
  line L198 (38.5617, -75.6473) -> (38.3121, -74.8305)
  line L199 (38.3121, -74.8305) -> (37.0544, -74.8305)
  line L200 (37.0544, -74.8305) -> (36.8016, -75.6473)
  point P0 (0, 0)
  dimension "d46" = 1.5989
  dimension "d47" = 1.5989
  constraints: 402 end point, 50 centre point, 20 point on circle, 810 other
  measures "d46" radial gap between concentric circles of A11 A0
  measures "d47" distance between parallel lines of L0 L1
extrude "Extrusion3" add sketch "Sketch3" against normal blind 2 contours A0 L0 A1 L22
extrude "Extrusion4" cut sketch "Sketch1" along normal blind 2 contours L40 A26 L41 A27 L42 A28 L43 A25
extrude "Extrusion5" cut sketch "Sketch2" against normal blind 1
extrude "Extrusion6" cut sketch "Sketch1" along normal through all contours L49 L48 L47 L46
fillet "Fillet2" radius 1.5 4 edges at (-46.1888, 1, 36) (27.2951, 1, 36) (27.2951, 1, 63.7839) (-46.1888, 1, 63.7839)
equation "\"d35\" = d34"
equation "\"d47\" = d46"
body "Solid1"
